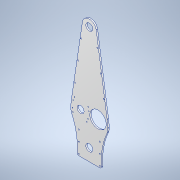
# Autodesk Inventor part: 関節3_側板1
Saved by Autodesk Inventor 2021 (Build 250183000, 183)
## iProperties
Created: 2022-02-02
Part Number: 関節3_側板1
Material: アルミニウム 6061
Document SubType Name: Modeling
Designer: hirohumi
Density: 2.7 g/cm^3
Appearance: アルミニウム - フラット
Author: hirohumi
Autodesk Inventor part; units mm, degrees
ref_plane "YZ Plane" through (0, 0, 0) normal (1, 0, 0) x (0, 1, 0)
ref_plane "XZ Plane" through (0, 0, 0) normal (0, 1, 0) x (-1, 0, 0)
ref_plane "XY Plane" through (0, 0, 0) normal (0, 0, 1) x (1, 0, 0)
sketch "スケッチ1" plane through (0, 0, 0) normal (0, 0, 1) x (1, 0, 0)
  circle A0 centre (0, 0) radius 10
  circle A1 centre (0, 0) radius 52 construction
  line L0 (30, 30) -> (-30, 30) construction
  line L1 (-30, 30) -> (-30, -30) construction
  line L2 (-30, -30) -> (30, -30) construction
  line L3 (30, -30) -> (30, 30) construction
  line L4 (30, 30) -> (-30, -30) construction
  line L5 (-30, 30) -> (30, -30) construction
  circle A2 centre (-30, 30) radius 1.6
  circle A3 centre (-30, 0) radius 1.6
  circle A4 centre (-30, -30) radius 1.6
  circle A5 centre (30, 30) radius 1.6
  circle A6 centre (30, 0) radius 1.6
  circle A7 centre (30, -30) radius 1.6
  circle A8 centre (-24.9956, 82.7025) radius 23.5 construction
  circle A9 centre (0, 0) radius 57 construction
  circle A10 centre (-24.9956, 82.7025) radius 10
  circle A11 centre (0, 300) radius 10
  line L6 (0, 300) -> (-24.9956, 82.7025) construction
  line L7 (-1.5003, 90.0658) -> (-46.2055, 95.2082) construction
  line L8 (-46.2055, 95.2082) -> (-48.491, 75.3392) construction
  line L9 (-48.491, 75.3392) -> (-3.7858, 70.1968) construction
  line L10 (-3.7858, 70.1968) -> (-1.5003, 90.0658) construction
  line L11 (-1.5003, 90.0658) -> (-48.491, 75.3392) construction
  line L12 (-46.2055, 95.2082) -> (-3.7858, 70.1968) construction
  line L13 (-2.8411, 100.286) -> (-42.5791, 104.857) construction
  line L14 (-42.5791, 104.857) -> (-47.1501, 65.119) construction
  line L15 (-47.1501, 65.119) -> (-7.4122, 60.548) construction
  line L16 (-7.4122, 60.548) -> (-2.8411, 100.286) construction
  line L17 (-2.8411, 100.286) -> (-47.1501, 65.119) construction
  line L18 (-42.5791, 104.857) -> (-7.4122, 60.548) construction
  circle A12 centre (-42.5791, 104.857) radius 1.25
  circle A13 centre (-46.2055, 95.2082) radius 1.25
  circle A14 centre (-48.491, 75.3392) radius 1.25
  circle A15 centre (-47.1501, 65.119) radius 1.25
  circle A16 centre (-2.8411, 100.286) radius 1.25
  circle A17 centre (-1.5003, 90.0658) radius 1.25
  circle A18 centre (-3.7858, 70.1968) radius 1.25
  circle A19 centre (-7.4122, 60.548) radius 1.25
  circle A20 centre (-1.5003, 90.0658) radius 4 construction
  circle A21 centre (-3.7858, 70.1968) radius 4 construction
  line L19 (0, 0) -> (0, 174.5579) construction
  circle A22 centre (24.9956, 82.7025) radius 23.5
  circle A23 centre (-7.4122, 60.548) radius 4 construction
  arc A24 (0, 320) -> (-19.7742, 302.9966) centre (0, 300) ccw
  arc A25 (-51.149, 95.9573) -> (-51.1727, 95.7796) centre (-46.2055, 95.2082) ccw
  arc A26 (-53.4582, 75.9106) -> (-53.4485, 74.6888) centre (-48.491, 75.3392) ccw
  arc A27 (-52.1076, 64.4686) -> (-51.6826, 63.0079) centre (-47.1501, 65.119) ccw
  arc A28 (-34.9844, -29.6047) -> (-30, -35) centre (-30, -30) ccw
  line L20 (-51.1727, 95.7796) -> (-53.4582, 75.9106)
  line L21 (-53.4485, 74.6888) -> (-52.1076, 64.4686)
  arc A29 (-34.9844, -29.6047) -> (-51.6826, 63.0079) centre (-219.1586, -15) ccw
  arc A30 (-31.6722, 4.7121) -> (-34.6924, -1.7267) centre (-30, 0) ccw construction
  line L22 (-19.7742, 302.9966) -> (-51.149, 95.9573)
  line L23 (-30, -35) -> (0, -35)
  circle A31 centre (-23.2557, 260) radius 1.6
  circle A32 centre (-41.2353, 141.3546) radius 1.6
  line L24 (-23.2557, 260) -> (-41.2353, 141.3546) construction
  circle A33 centre (-32.2455, 200.6773) radius 1.6
  arc A34 (19.7742, 302.9966) -> (0, 320) centre (0, 300) ccw
  arc A35 (51.1727, 95.7796) -> (51.149, 95.9573) centre (46.2055, 95.2082) ccw
  arc A36 (53.4485, 74.6888) -> (53.4582, 75.9106) centre (48.491, 75.3392) ccw
  arc A37 (51.6826, 63.0079) -> (52.1076, 64.4686) centre (47.1501, 65.119) ccw
  arc A38 (30, -35) -> (34.9844, -29.6047) centre (30, -30) ccw
  line L25 (51.1727, 95.7796) -> (53.4582, 75.9106)
  line L26 (53.4485, 74.6888) -> (52.1076, 64.4686)
  arc A39 (51.6826, 63.0079) -> (34.9844, -29.6047) centre (219.1586, -15) ccw
  line L27 (19.7742, 302.9966) -> (51.149, 95.9573)
  line L28 (30, -35) -> (0, -35)
  circle A40 centre (23.2557, 260) radius 1.6
  circle A41 centre (41.2353, 141.3546) radius 1.6
  circle A42 centre (32.2455, 200.6773) radius 1.6
  dimension "d0" = 20
  dimension "d1" = 104
  dimension "d2" = 60
  dimension "d3" = 60
  dimension "d4" = 3.2
  dimension "d5" = 3.2
  dimension "d6" = 3.2
  dimension "d7" = 3.2
  dimension "d8" = 3.2
  dimension "d9" = 3.2
  dimension "d10" = 47
  dimension "d12" = 5
  dimension "d13" = 20
  dimension "d14" = 20
  dimension "d15" = 300
  dimension "d16" = 20
  dimension "d17" = 45
  dimension "d18" = 40
  dimension "d19" = 40
  dimension "d20" = 2.5
  dimension "d21" = 2.5
  dimension "d22" = 2.5
  dimension "d23" = 2.5
  dimension "d24" = 2.5
  dimension "d25" = 2.5
  dimension "d26" = 2.5
  dimension "d27" = 2.5
  dimension "d28" = 8
  dimension "d29" = 8
  dimension "d30" = 8
  dimension "d31" = 20
  dimension "d33" = 5
  dimension "d34" = 5
  dimension "d35" = 5
  dimension "d36" = 5
  dimension "d37" = 5
  dimension "d38" = 3.2
  dimension "d39" = 3.2
  dimension "d40" = 3
  dimension "d41" = 120
  dimension "d42" = 40
  dimension "d43" = 3.2
  constraints: 58 end point, 43 centre point, 26 point on circle, 24 coincident, 18 symmetric about line, 12 tangent, 10 midpoint, 7 parallel, 5 perpendicular, 2 horizontal, 2 vertical alignment, 1 vertical, 10 other
  measures "d0" diameter of A0
  measures "d1" diameter of A1
  measures "d2" distance of L2.end L1.end
  measures "d3" distance of L1.end L0.end
  measures "d4" diameter of A2
  measures "d5" diameter of A3
  measures "d6" diameter of A4
  measures "d7" diameter of A5
  measures "d8" diameter of A6
  measures "d9" diameter of A7
  measures "d10" diameter of A8
  measures "d12" radial gap between concentric circles of A1 A9
  measures "d13" diameter of A10
  measures "d14" diameter of A11
  measures "d15" distance of point (0, 0) L6.start
  measures "d16" distance of L7.end L8.end
  measures "d17" distance of L8.end L9.end
  measures "d18" distance of L14.end L15.end
  measures "d19" distance of L13.end L14.end
  measures "d20" diameter of A12
  measures "d21" diameter of A13
  measures "d22" diameter of A14
  measures "d23" diameter of A15
  measures "d24" diameter of A16
  measures "d25" diameter of A17
  measures "d26" diameter of A18
  measures "d27" diameter of A19
  measures "d28" diameter of A20
  measures "d29" diameter of A21
  measures "d30" diameter of A23
  measures "d31" radius of A24
  measures "d33" radius of A25
  measures "d34" radius of A26
  measures "d35" radius of A27
  measures "d36" radius of A28
  measures "d37" radius of A30
  measures "d38" diameter of A31
  measures "d39" diameter of A32
  measures "d40" distance between parallel lines of L22 L24
  measures "d41" distance of L24.start L24.end
  measures "d42" vertical distance of L24.start L6.start
  measures "d43" diameter of A33
extrude "押し出し1" add sketch "スケッチ1" along normal blind 4
